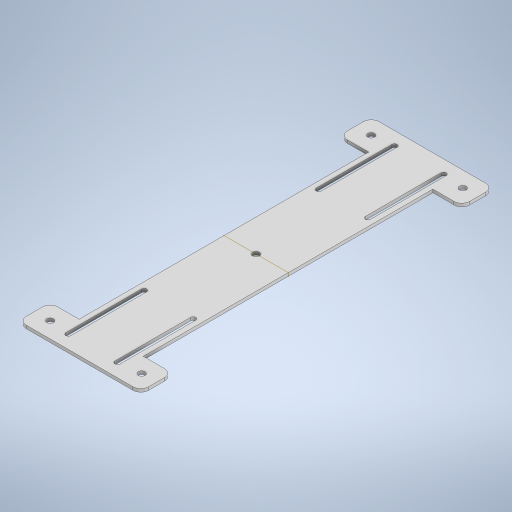
# Autodesk Inventor part: Motor Attachment 2.0
Saved by Autodesk Inventor 2024 (Build 280153000, 153)
## iProperties
Created: 2023-10-21
Part Number: Motor Attachment 2.0
Material: Generic
Document SubType Name: Modeling
Designer: olson
Density: 1 g/cm^3
Appearance: Default
Author: olson
Autodesk Inventor part; units mm, degrees
ref_plane "YZ Plane" through (0, 0, 0) normal (1, 0, 0) x (0, 1, 0)
ref_plane "XZ Plane" through (0, 0, 0) normal (0, 1, 0) x (-1, 0, 0)
ref_plane "XY Plane" through (0, 0, 0) normal (0, 0, 1) x (1, 0, 0)
sketch "Sketch1" plane through (0, 0, 0) normal (0, 1, 0) x (-1, 0, 0)
  line L0 (0, 0) -> (-37.6, 0)
  line L1 (-37.6, -20) -> (-37.6, -51.2)
  line L2 (-37.6, -51.2) -> (0, -51.2)
  line L3 (0, -51.2) -> (0, -20)
  line L4 (-18.8, 0) -> (-1.65, 0)
  line L5 (-1.65, 0) -> (-23.35, 0)
  line L6 (-18.8, 0) -> (5.35, 0)
  line L7 (5.35, 0) -> (-25.85, 0)
  line L8 (-18.8, 0) -> (-3.2, 0)
  line L9 (-3.2, 0) -> (-34.4, 0)
  arc A0 (-32.8, -8.4) -> (-36, -8.4) centre (-34.4, -8.4) ccw
  arc A1 (-36, -46.5) -> (-32.8, -46.5) centre (-34.4, -46.5) ccw
  arc A2 (-1.6, -8.4) -> (-4.8, -8.4) centre (-3.2, -8.4) ccw
  arc A3 (-4.8, -46.5) -> (-1.6, -46.5) centre (-3.2, -46.5) ccw
  line L10 (0, 0) -> (0, -20)
  line L11 (0, -20) -> (20, -20)
  line L12 (20, -20) -> (20, 0)
  line L13 (20, 0) -> (0, 0)
  line L14 (-37.6, -20) -> (-57.6, -20)
  line L15 (-57.6, -20) -> (-57.6, 0)
  line L16 (-57.6, 0) -> (-37.6, 0)
  line L17 (-1.6, -46.5) -> (-1.6, -8.4)
  line L18 (-4.8, -8.4) -> (-4.8, -46.5)
  line L19 (-32.8, -46.5) -> (-32.8, -8.4)
  line L20 (-36, -8.4) -> (-36, -46.5)
  point P0 (5.35, 0)
  dimension "d0" = 37.6
  dimension "d1" = 51.2
  dimension "d41" = 15.6
  dimension "d42" = 31.2
  dimension "d50" = 3.2
  dimension "d56" = 3.2
  dimension "d57" = 3.2
  dimension "d63" = 3.2
  dimension "d67" = 8.4
  dimension "d77" = 8.4
  dimension "d81" = 20
  dimension "d82" = 20
  dimension "d83" = 20
  constraints: 42 end point, 9 point on line, 8 point on circle, 6 perpendicular, 6 tangent, 4 centre point, 2 parallel, 1 horizontal, 1 midpoint
  measures "d0" distance of L2.end L1.end
  measures "d1" distance of L1.end L0.end
  measures "d41" distance of L4.start L8.end
  measures "d42" distance of L8.end L9.end
  measures "d50" diameter of A0
  measures "d56" diameter of A1
  measures "d57" diameter of A2
  measures "d63" diameter of A3
  measures "d67" distance of L8.end A2.centre
  measures "d77" distance of L9.end A0.centre
  measures "d81" distance of L3.end L0.start
  measures "d82" distance of L3.end L11.end
  measures "d83" distance of L1.start L14.end
extrude "Extrusion3" add sketch "Sketch1" along normal blind 2
sketch "Sketch2" plane through (0, 2, 0) normal (0, 1, 0) x (1, 0, 0)
  circle A0 centre (-10, 10) radius 2.125
  line L0 (-20, 0) -> (57.6, 0) projected
  line L1 (38.17, 0) -> (48.17, 0)
  circle A1 centre (48.17, 10) radius 2.125
  point P0 (0, 0)
  dimension "d85" = 4.25
  dimension "d86" = 10
  dimension "d88" = 4.25
  constraints: 2 centre point, 2 end point, 2 point on line
  measures "d85" diameter of A0
  measures "d86" distance of L1.start L1.end
  measures "d88" diameter of A1
extrude "Extrusion4" cut sketch "Sketch2" against normal blind 2
fillet "Fillet3" radius 5 4 edges at (57.6, 1, -20) (57.6, 1, 0) (-20, 1, 0) (-20, 1, -20)
ref_plane "Work Plane2" through (37.6, 0, -112) normal (0, 0, -1) x (-1, 0, 0)
mirror "Mirror2" about plane through (37.6, 0, -112) normal (0, 0, -1)
sketch "Sketch5" plane through (0, 0, 0) normal (0, 1, 0) x (-1, 0, 0)
  line L0 (-37.6, -172.8) -> (0, -172.8)
  line L1 (0, -51.2) -> (-37.6, -51.2)
  line L2 (20, -112) -> (20, -102)
  line L3 (20, -102) -> (0, -102)
  line L4 (20, -112) -> (20, -122)
  line L5 (20, -122) -> (0, -122)
  line L6 (-37.6, -122) -> (-57.6, -122)
  line L7 (-57.6, -122) -> (-57.6, -102)
  line L8 (-57.6, -102) -> (-37.6, -102)
  line L9 (-37.6, -51.2) -> (-37.6, -102)
  line L10 (-37.6, -122) -> (-37.6, -172.8)
  line L11 (0, -172.8) -> (0, -122)
  line L12 (0, -102) -> (0, -51.2)
  circle A0 centre (10, -112) radius 2.125
  circle A1 centre (-47.6, -112) radius 2.125
  point P0 (0, 0)
  dimension "d95" = 10
  dimension "d96" = 10
  dimension "d97" = 20
  dimension "d98" = 4.25
  dimension "d99" = 4.25
  constraints: 26 end point, 11 perpendicular, 5 point on line, 2 centre point
  measures "d95" distance of L2.start L2.end
  measures "d96" distance of L2.start L4.end
  measures "d97" distance of L6.start L6.end
  measures "d98" diameter of A0
  measures "d99" diameter of A1
extrude "Extrusion5" add sketch "Sketch5" along normal blind 2
fillet "Fillet4" radius 5 4 edges at (57.6, 1, -122) (57.6, 1, -102) (-20, 1, -122) (-20, 1, -102)
sketch "Sketch6" plane through (0, 2, 0) normal (0, 1, 0) x (1, 0, 0)
  arc A0 (4.8, 46.5) -> (1.6, 46.5) centre (3.2, 46.5) ccw projected
  line L0 (3.2, 46.5) -> (13.2, 46.5) construction
  arc A1 (36, 56.5) -> (32.8, 56.5) centre (34.4, 56.5) ccw
  arc A2 (3.2, 54.9) -> (1.6, 56.5) centre (3.2, 56.5) ccw
  arc A3 (36, 46.5) -> (32.8, 46.5) centre (34.4, 46.5) ccw projected
  line L1 (36, 46.5) -> (36, 56.5)
  line L2 (32.8, 46.5) -> (32.8, 56.5)
  line L3 (4.8, 46.5) -> (4.8, 56.5)
  line L4 (1.6, 46.5) -> (1.6, 56.5)
  circle A4 centre (34.4, 46.5) radius 1.6
  circle A5 centre (3.2, 46.5) radius 1.6
  point P0 (0, 0)
  constraints: 10 end point, 6 point on circle, 4 centre point, 2 coincident, 2 tangent, 1 horizontal, 1 parallel
extrude "Extrusion6" cut sketch "Sketch6" against normal blind 2 contours A0 L4 A2 L3 | L1 A3 L2 A1
sketch "Sketch7" plane through (0, 2, 0) normal (0, 1, 0) x (1, 0, 0)
  arc A0 (1.6, 177.5) -> (4.8, 177.5) centre (3.2, 177.5) ccw projected
  arc A1 (1.6, 167.5) -> (4.8, 167.5) centre (3.2, 167.5) ccw
  arc A2 (32.8, 167.5) -> (36, 167.5) centre (34.4, 167.5) ccw
  arc A3 (32.8, 177.5) -> (36, 177.5) centre (34.4, 177.5) ccw projected
  line L0 (36, 177.5) -> (36, 167.5)
  line L1 (32.8, 177.5) -> (32.8, 167.5)
  line L2 (1.6, 177.5) -> (1.6, 167.5)
  line L3 (4.8, 167.5) -> (4.8, 177.5)
  arc A4 (1.6, 177.5) -> (4.8, 177.5) centre (3.2, 177.5) ccw
  arc A5 (32.8, 177.5) -> (36, 177.5) centre (34.4, 177.5) ccw
  point P0 (0, 0)
  constraints: 8 end point, 8 point on circle, 4 centre point, 3 tangent, 2 coincident, 2 concentric, 1 parallel
extrude "Extrusion7" cut sketch "Sketch7" against normal blind 2
sketch "Sketch8" plane through (0, 2, 0) normal (0, 1, 0) x (1, 0, 0)
  line L0 (0, 122) -> (-15, 122) projected
  line L1 (0, 122) -> (-20, 122)
  line L2 (-20, 122) -> (-20, 102)
  line L3 (-20, 102) -> (0, 102)
  line L4 (0, 102) -> (0, 122)
  point P0 (0, 0)
  constraints: 8 end point, 2 parallel, 1 horizontal, 1 perpendicular
extrude "Extrusion8" cut sketch "Sketch8" against normal blind 2
sketch "Sketch9" plane through (0, 2, 0) normal (0, 1, 0) x (1, 0, 0)
  line L0 (52.6, 122) -> (37.6, 122) projected
  line L1 (37.6, 122) -> (57.6, 122)
  line L2 (57.6, 122) -> (57.6, 102)
  line L3 (57.6, 102) -> (37.6, 102)
  line L4 (37.6, 102) -> (37.6, 122)
  point P0 (0, 0)
  constraints: 8 end point, 2 parallel, 1 horizontal, 1 perpendicular
extrude "Extrusion9" cut sketch "Sketch9" against normal blind 2
sketch "Sketch10" plane through (0, 2, 0) normal (0, 1, 0) x (1, 0, 0)
  line L0 (0, 0) -> (18.8, 0)
  line L1 (-15, 0) -> (52.6, 0) projected
  line L2 (18.8, 0) -> (18.8, 112)
  circle A0 centre (18.8, 112) radius 2.125
  dimension "d114" = 112
  dimension "d115" = 4.25
  constraints: 4 end point, 1 centre point, 1 coincident, 1 midpoint, 1 perpendicular
  measures "d114" distance of L0.end L2.end
  measures "d115" diameter of A0
extrude "Extrusion10" cut sketch "Sketch10" against normal blind 2
sketch "Sketch11" plane through (0, 2, 0) normal (0, 1, 0) x (1, 0, 0)
  line L0 (0, 20) -> (0, 204) projected
  line L1 (0, 204) -> (-15, 204) projected
  line L2 (0, 20) -> (-1.6, 20)
  line L3 (-1.6, 20) -> (-1.6, 204)
  line L4 (-1.6, 204) -> (0, 204)
  line L5 (0, 204) -> (0, 20)
  line L6 (37.6, 20) -> (37.6, 204) projected
  line L7 (37.6, 204) -> (39.2, 204)
  line L8 (39.2, 204) -> (39.2, 20)
  line L9 (39.2, 20) -> (37.6, 20)
  line L10 (37.6, 20) -> (37.6, 204)
  point P0 (0, 0)
  dimension "d118" = 1.6
  dimension "d119" = 1.6
  constraints: 16 end point, 4 parallel, 2 horizontal, 2 perpendicular, 2 point on line
  measures "d118" distance of L3.end L4.end
  measures "d119" distance of L8.end L9.end
extrude "Extrusion11" add sketch "Sketch11" against normal blind 2
body "Solid3"
